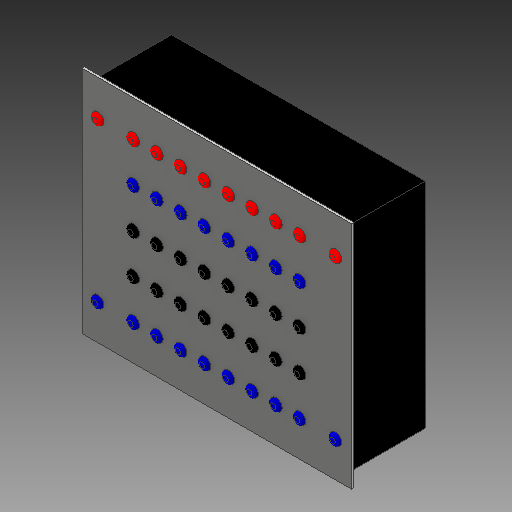
# Autodesk Inventor part: Uni
Saved by Autodesk Inventor 2019 (Build 230136000, 136)
## iProperties
Created: 2019-04-25
Part Number: Uni
Material: Generic
Document SubType Name: Modeling
Designer: felix
Density: 1 g/cm^3
Appearance: Default
Mass: 8960.63 g
Surface Area: 3234.01 cm^2
Volume: 8960.63 cm^3
Author: felix
Autodesk Inventor part; units mm, degrees
ref_plane "YZ Plane" through (0, 0, 0) normal (1, 0, 0) x (0, 1, 0)
ref_plane "XZ Plane" through (0, 0, 0) normal (0, 1, 0) x (-1, 0, 0)
ref_plane "XY Plane" through (0, 0, 0) normal (0, 0, 1) x (1, 0, 0)
sketch "Sketch1" plane through (0, 0, 0) normal (0, 0, 1) x (1, 0, 0)
  line L0 (0, 0) -> (-320, 0)
  line L1 (-320, 0) -> (-320, 270)
  line L2 (-320, 270) -> (0, 270)
  line L3 (0, 270) -> (0, 0)
  dimension "d0" = 320
  dimension "d1" = 270
  constraints: 8 end point, 2 parallel, 1 horizontal, 1 perpendicular
  measures "d0" distance of L0.start L0.end
  measures "d1" distance between parallel lines of L0 L2
extrude "Extrusion1" add sketch "Sketch1" along normal blind 100
sketch "Sketch2" plane through (0, 0, 100) normal (0, 0, 1) x (1, 0, 0)
  line L0 (10, -10) -> (-330, -10)
  line L1 (-330, -10) -> (-330, 280)
  line L2 (-330, 280) -> (10, 280)
  line L3 (10, 280) -> (10, -10)
  point P0 (0, 0)
  dimension "d4" = 340
  dimension "d5" = 290
  dimension "d6" = 10
  dimension "d7" = 10
  constraints: 8 end point, 2 parallel, 1 horizontal, 1 perpendicular
  measures "d4" distance of L0.start L0.end
  measures "d5" distance of L2.end L0.start
  measures "d6" horizontal distance of L0.start point (0, 0)
  measures "d7" horizontal distance of L0.start point (0, 0)
extrude "Extrusion2" add sketch "Sketch2" along normal blind 3
sketch "Sketch3" plane through (0, 0, 103) normal (0, 0, 1) x (1, 0, 0)
  circle A0 centre (-265, 85) radius 7.5
  line L0 (0, 0) -> (0, 270) projected
  circle A1 centre (-265, 135) radius 7.5
  circle A2 centre (-265, 185) radius 7.5
  circle A3 centre (-265, 235) radius 7.5
  circle A4 centre (-265, 35) radius 7.5
  circle A5 centre (-310, 35) radius 7.5
  circle A6 centre (-310, 235) radius 7.5
  line L1 (-320, 0) -> (0, 0) projected
  circle A7 centre (-235, 235) radius 7.5
  circle A8 centre (-235, 185) radius 7.5
  circle A9 centre (-235, 85) radius 7.5
  circle A10 centre (-235, 135) radius 7.5
  circle A11 centre (-235, 35) radius 7.5
  circle A12 centre (-205, 235) radius 7.5
  circle A13 centre (-205, 185) radius 7.5
  circle A14 centre (-205, 85) radius 7.5
  circle A15 centre (-205, 135) radius 7.5
  circle A16 centre (-205, 35) radius 7.5
  circle A17 centre (-175, 235) radius 7.5
  circle A18 centre (-175, 185) radius 7.5
  circle A19 centre (-175, 85) radius 7.5
  circle A20 centre (-175, 135) radius 7.5
  circle A21 centre (-175, 35) radius 7.5
  circle A22 centre (-145, 235) radius 7.5
  circle A23 centre (-145, 185) radius 7.5
  circle A24 centre (-145, 85) radius 7.5
  circle A25 centre (-145, 135) radius 7.5
  circle A26 centre (-145, 35) radius 7.5
  circle A27 centre (-115, 235) radius 7.5
  circle A28 centre (-115, 185) radius 7.5
  circle A29 centre (-115, 85) radius 7.5
  circle A30 centre (-115, 135) radius 7.5
  circle A31 centre (-115, 35) radius 7.5
  circle A32 centre (-85, 235) radius 7.5
  circle A33 centre (-85, 185) radius 7.5
  circle A34 centre (-85, 85) radius 7.5
  circle A35 centre (-85, 135) radius 7.5
  circle A36 centre (-85, 35) radius 7.5
  circle A37 centre (-55, 235) radius 7.5
  circle A38 centre (-55, 185) radius 7.5
  circle A39 centre (-55, 85) radius 7.5
  circle A40 centre (-55, 135) radius 7.5
  circle A41 centre (-55, 35) radius 7.5
  circle A42 centre (-10, 235) radius 7.5
  circle A43 centre (-10, 35) radius 7.5
  point P0 (0, 180)
  point P1 (-230, 0)
  dimension "d11" = 15
  dimension "d12" = 265
  dimension "d13" = 85
  dimension "d14" = 135
  dimension "d16" = 185
  dimension "d17" = 235
  dimension "d18" = 35
  dimension "d19" = 310
  dimension "d22" = 30
  dimension "d27" = 10
  constraints: 44 centre point, 8 equal radius, 6 vertical alignment, 4 horizontal alignment, 1 horizontal, 70 other
  measures "d11" diameter of A0
  measures "d12" distance from line of L0 A0.centre
  measures "d13" vertical distance of L0.start A0.centre
  measures "d14" vertical distance of L0.start A1.centre
  measures "d16" vertical distance of L0.start A2.centre
  measures "d17" vertical distance of L0.start A3.centre
  measures "d18" vertical distance of L0.start A4.centre
  measures "d19" horizontal distance of L0.start A5.centre
  measures "d22" distance of A3.centre A7.centre
  measures "d27" horizontal distance of L0.start A42.centre
extrude "Extrusion3" add sketch "Sketch3" along normal blind 4
fillet "Fillet1" radius 4 44 edges at (-317.5, 235, 107) (-272.5, 235, 107) (-242.5, 235, 107) (-212.5, 235, 107) (-182.5, 235, 107) (-152.5, 235, 107) (-122.5, 235, 107) (-92.5, 235, 107) (-62.5, 235, 107) (-17.5, 235, 107) (-272.5, 185, 107) (-242.5, 185, 107) (-212.5, 185, 107) (-182.5, 185, 107) (-152.5, 185, 107) (-122.5, 185, 107) (-92.5, 185, 107) (-62.5, 185, 107) (-62.5, 85, 107) (-92.5, 85, 107) (-122.5, 85, 107) (-152.5, 85, 107) (-182.5, 85, 107) (-212.5, 85, 107) (-242.5, 85, 107) (-272.5, 85, 107) (-272.5, 135, 107) (-242.5, 135, 107) (-212.5, 135, 107) (-182.5, 135, 107) (-152.5, 135, 107) (-122.5, 135, 107) (-92.5, 135, 107) (-62.5, 135, 107) (-317.5, 35, 107) (-272.5, 35, 107) (-242.5, 35, 107) (-212.5, 35, 107) (-182.5, 35, 107) (-152.5, 35, 107) (-122.5, 35, 107) (-92.5, 35, 107) (-62.5, 35, 107) (-17.5, 35, 107)
body "Solid1"
